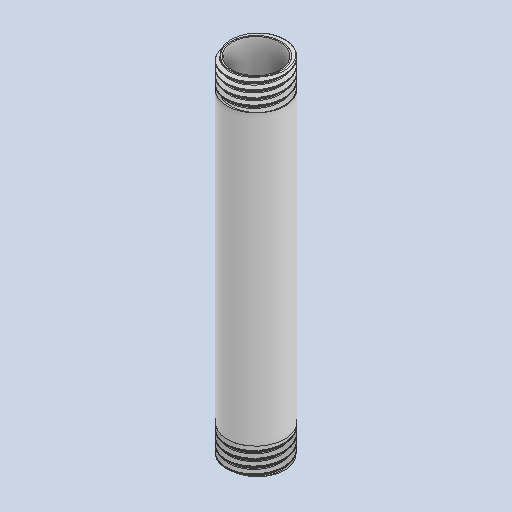
# Autodesk Inventor part: OutputFile
Saved by Autodesk Inventor 2023.1 (Build 271208000, 208)
## iProperties
Created: 2023-11-18
Part Number: OutputFile
Material: Generic
Document SubType Name: Modeling
Designer: danie
Density: 1 g/cm^3
Appearance: Default
Mass: 38.8772 g
Surface Area: 315.337 cm^2
Volume: 38.8772 cm^3
Author: danie
Autodesk Inventor part; units mm, degrees
ref_plane "YZ Plane" through (0, 0, 0) normal (1, 0, 0) x (0, 1, 0)
ref_plane "XZ Plane" through (0, 0, 0) normal (0, 1, 0) x (-1, 0, 0)
ref_plane "XY Plane" through (0, 0, 0) normal (0, 0, 1) x (1, 0, 0)
sketch "Sketch1" plane through (0, 0, 0) normal (0, 1, 0) x (-1, 0, 0)
  circle A0 centre (0, 0) radius 15
  circle A1 centre (0, 0) radius 12.5
  dimension "d0" = 30
  dimension "d1" = 25
  constraints: 2 centre point, 2 coincident
  measures "d0" diameter of A0
  measures "d1" diameter of A1
extrude "Extrusion1" add sketch "Sketch1" along normal blind 180
thread "Thread1" size "M30x3.5" class "6g" standard "ANSI Metric M Profile" length 15
thread "Thread2" size "M30x3.5" class "6g" standard "ANSI Metric M Profile" length 15
sketch "Sketch3" plane through (0, 0, 0) normal (-1, 0, 0) x (0, 0, 1)
  line L0 (15, 0) -> (15, 15)
  line L1 (15, 15) -> (13.1056, 15)
  line L2 (13.1056, 15) -> (13.1056, 0)
  line L3 (13.1056, 0) -> (15, 0)
  line L4 (0, -40.4625) -> (0, 216.7437) projected
  constraints: 8 end point
revolve "Revolution1" cut sketch "Sketch3" angle 360 about axis through (0, 0, 0) along (0, 1, 0)
sketch "Sketch4" plane through (0, 0, 0) normal (-1, 0, 0) x (0, 0, 1)
  line L0 (15, 0) -> (15, 15)
  line L1 (15, 15) -> (13.1056, 15)
  line L2 (13.1056, 15) -> (13.1056, 0)
  line L3 (13.1056, 0) -> (15, 0)
  line L4 (0, -40.4625) -> (0, 216.7437) projected
  constraints: 8 end point
revolve "Revolution2" add sketch "Sketch4" angle 360 about axis through (0, 0, 0) along (0, 1, 0) separate body
sketch "Sketch2" plane through (0, 0, 0) normal (1, 0, 0) x (0, 1, 0)
  line L0 (-1.75, -12.3478) -> (-2.3138, -13.3243) construction
  line L1 (-1.75, -12.3478) -> (-1.1862, -13.3243) construction
  line L2 (-1.75, -12.3478) -> (-1.75, -13.1056) construction
  line L3 (-2.1875, -13.1056) -> (-1.9349, -13.1056) construction
  line L4 (0, -15.3789) -> (0.2187, -15) construction
  line L5 (-3.5, -15.3789) -> (-3.7187, -15) construction
  line L6 (-3.7187, -15) -> (-3.5, -15) construction
  line L7 (-3.2813, -15) -> (-3.5, -15.3789) construction
  arc A0 (-1.9349, -13.1056) -> (-2.3138, -13.3243) centre (-1.9349, -13.5431) ccw
  arc A1 (-1.1862, -13.3243) -> (-1.5651, -13.1056) centre (-1.5651, -13.5431) ccw
  line L8 (0, -15.3789) -> (0, -15) construction
  line L9 (-3.5, -15.3789) -> (-3.5, -15) construction
  arc A2 (-0.2819, -14.8906) -> (-0.0925, -15) centre (-0.0925, -14.7812) ccw
  line L10 (-1.1862, -13.3243) -> (-0.2819, -14.8906)
  line L11 (-1.9349, -13.1056) -> (-1.5651, -13.1056)
  line L12 (-2.3138, -13.3243) -> (-3.2181, -14.8906)
  line L13 (-0.0925, -15) -> (0, -15) construction
  line L14 (0, -15) -> (0.2187, -15) construction
  arc A3 (-3.4075, -15) -> (-3.2181, -14.8906) centre (-3.4075, -14.7812) ccw
  line L15 (-3.2181, -14.8906) -> (-3.2813, -15) construction
  line L16 (-3.5, -15) -> (-3.4075, -15) construction
  line L17 (-3.4075, -15) -> (-0.0925, -15)
  line L18 (0, 0) -> (0.4413, 0)
  line L19 (0, 0) -> (0, 0.419)
  line L20 (0, -15.3789) -> (-0.2819, -14.8906) construction
  dimension "d8" = 0.7578
  dimension "d9" = 0.4375
  dimension "d10" = 0.2188
  dimension "d11" = 0.3789
  dimension "d12" = 3.5
  dimension "Sketch2_MajorRadius" = 15
  dimension "d14" = 60
  dimension "Sketch2_ThreadOffset" = 0
  dimension "Sketch2_MinorRadius" = 13.1056
  constraints: 42 end point, 17 tangent, 8 point on circle, 6 parallel, 5 collinear, 4 centre point, 3 point on line, 3 vertical, 2 equal radius, 2 horizontal, 2 perpendicular, 1 equal length, 1 midpoint, 4 other
  measures "d8" distance from line of L0.start L3
  measures "d9" radius of A0
  measures "d10" radius of A2
  measures "d11" distance from line of L14 L4.start
  measures "d12" distance between parallel lines of L8 L9
  measures "Sketch2_MajorRadius" distance between parallel lines of L14 L18
  measures "d14" angle of L10 L12
  measures "Sketch2_ThreadOffset" distance between parallel lines of L19 L8
  measures "Sketch2_MinorRadius" distance between parallel lines of L18 L11
coil "Coil1" sketch "Sketch2" operation cut axis through (0, 0, 0) along (0, 1, 0) pitch 3.5035 turns 6.279435 hand right bodies 2
sketch "Sketch6" plane through (0, 180, 0) normal (1, 0, 0) x (0, 0, 1)
  line L0 (15, 0) -> (15, 15)
  line L1 (15, 15) -> (13.1056, 15)
  line L2 (13.1056, 15) -> (13.1056, 0)
  line L3 (13.1056, 0) -> (15, 0)
  line L4 (0, -40.6434) -> (0, 217.8289) projected
  constraints: 8 end point
revolve "Revolution3" cut sketch "Sketch6" angle 360 about axis through (0, 180, 0) along (0, -1, 0) bodies 1
sketch "Sketch7" plane through (0, 180, 0) normal (1, 0, 0) x (0, 0, 1)
  line L0 (15, 0) -> (15, 15)
  line L1 (15, 15) -> (13.1056, 15)
  line L2 (13.1056, 15) -> (13.1056, 0)
  line L3 (13.1056, 0) -> (15, 0)
  line L4 (0, -40.6434) -> (0, 217.8289) projected
  constraints: 8 end point
revolve "Revolution4" add sketch "Sketch7" angle 360 about axis through (0, 180, 0) along (0, -1, 0) separate body
sketch "Sketch5" plane through (0, 180, 0) normal (-1, 0, 0) x (0, -1, 0)
  line L0 (-1.75, -12.3478) -> (-2.3138, -13.3243) construction
  line L1 (-1.75, -12.3478) -> (-1.1862, -13.3243) construction
  line L2 (-1.75, -12.3478) -> (-1.75, -13.1056) construction
  line L3 (-2.1875, -13.1056) -> (-1.9349, -13.1056) construction
  line L4 (0, -15.3789) -> (0.2187, -15) construction
  line L5 (-3.5, -15.3789) -> (-3.7187, -15) construction
  line L6 (-3.7187, -15) -> (-3.5, -15) construction
  line L7 (-3.2813, -15) -> (-3.5, -15.3789) construction
  arc A0 (-1.9349, -13.1056) -> (-2.3138, -13.3243) centre (-1.9349, -13.5431) ccw
  arc A1 (-1.1862, -13.3243) -> (-1.5651, -13.1056) centre (-1.5651, -13.5431) ccw
  line L8 (0, -15.3789) -> (0, -15) construction
  line L9 (-3.5, -15.3789) -> (-3.5, -15) construction
  arc A2 (-0.2819, -14.8906) -> (-0.0925, -15) centre (-0.0925, -14.7812) ccw
  line L10 (-1.1862, -13.3243) -> (-0.2819, -14.8906)
  line L11 (-1.9349, -13.1056) -> (-1.5651, -13.1056)
  line L12 (-2.3138, -13.3243) -> (-3.2181, -14.8906)
  line L13 (-0.0925, -15) -> (0, -15) construction
  line L14 (0, -15) -> (0.2187, -15) construction
  arc A3 (-3.4075, -15) -> (-3.2181, -14.8906) centre (-3.4075, -14.7812) ccw
  line L15 (-3.2181, -14.8906) -> (-3.2813, -15) construction
  line L16 (-3.5, -15) -> (-3.4075, -15) construction
  line L17 (-3.4075, -15) -> (-0.0925, -15)
  line L18 (0, 0) -> (0.4413, 0)
  line L19 (0, 0) -> (0, 0.419)
  line L20 (0, -15.3789) -> (-0.2819, -14.8906) construction
  dimension "d30" = 0.7578
  dimension "d31" = 0.4375
  dimension "d32" = 0.2188
  dimension "d33" = 0.3789
  dimension "d34" = 3.5
  dimension "Sketch5_MajorRadius" = 15
  dimension "d36" = 60
  dimension "Sketch5_ThreadOffset" = 0
  dimension "Sketch5_MinorRadius" = 13.1056
  constraints: 42 end point, 17 tangent, 8 point on circle, 6 parallel, 5 collinear, 4 centre point, 3 point on line, 3 vertical, 2 equal radius, 2 horizontal, 2 perpendicular, 1 equal length, 1 midpoint, 4 other
  measures "d30" distance from line of L0.start L3
  measures "d31" radius of A0
  measures "d32" radius of A2
  measures "d33" distance from line of L14 L4.start
  measures "d34" distance between parallel lines of L8 L9
  measures "Sketch5_MajorRadius" distance between parallel lines of L14 L18
  measures "d36" angle of L10 L12
  measures "Sketch5_ThreadOffset" distance between parallel lines of L19 L8
  measures "Sketch5_MinorRadius" distance between parallel lines of L18 L11
coil "Coil2" sketch "Sketch5" operation cut axis through (0, 180, 0) along (0, -1, 0) pitch 3.5035 turns 6.279435 hand right bodies 3
equation "\"d8\" = 0.216506 * Sketch2_Pitch"
equation "\"d9\" = d17"
equation "\"d10\" = 0.0625 * Sketch2_Pitch"
equation "\"d11\" = 0.108253 * Sketch2_Pitch"
equation "\"d12\" = Sketch2_Pitch"
equation "\"d14\" = d19"
equation "\"d30\" = 0.216506 * Sketch5_Pitch"
equation "\"d31\" = d39"
equation "\"d32\" = 0.0625 * Sketch5_Pitch"
equation "\"d33\" = 0.108253 * Sketch5_Pitch"
equation "\"d34\" = Sketch5_Pitch"
equation "\"d36\" = d41"
equation "\"d17\" = 0.125 * Sketch2_Pitch"
equation "\"Sketch2_Pitch\" = 3.5"
equation "\"d19\" = 60deg"
equation "\"d39\" = 0.125 * Sketch5_Pitch"
equation "\"Sketch5_Pitch\" = 3.5"
equation "\"d41\" = 60deg"
body "Solid1"
body "Solid2"
body "Solid3"
